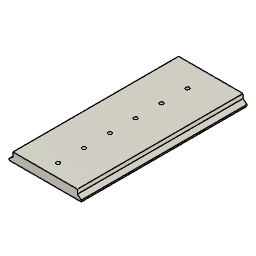
Fan Mount 50mm - BLANK_OLDV3_0 (Autodesk Fusion 360 design; units mm, degrees)
Autodesk Fusion 360 part; units mm, degrees
sketch "Sketch1" plane through (0, 0, 0) normal (0, 0, 1) x (1, 0, 0)
  line L0 (-27.9, 64) -> (27.9, 64)
  line L1 (27.9, 64) -> (27.9, -64)
  line L2 (27.9, -64) -> (-27.9, -64)
  line L3 (-27.9, -64) -> (-27.9, 64)
  line L4 (0, 76.2027) -> (0, 75)
  line L5 (0, 75) -> (0, -75) construction
  line L6 (-56.392, 0) -> (-53.853, 0)
  line L7 (-53.853, 0) -> (53.853, 0) construction
  point P0 (0, 64)
  point P1 (-27.9, 0)
  dimension "d44" = 150
  dimension "d45" = 128
  dimension "d46" = 55.8
  constraint horizontal L0
  constraint vertical L1
  constraint horizontal L2
  constraint vertical L3
  constraint midpoint L0 P0
  constraint midpoint L3 P1
  constraint vertical L4
  constraint parallel L4 L5
  constraint midpoint origin L5
  constraint perpendicular L3 L6
  constraint perpendicular L1 L7
  constraint midpoint origin L7
  constraint coincident P1 L7
  constraint coincident P0 L5
  measures "d44" distance of L4.end L5.end
  measures "d45" distance of L0.start L2.end
  measures "d46" distance of L0.start L0.end
extrude "Extrude1" add sketch "Sketch1" along normal blind 7
sketch "Sketch2" plane through (0, -64, 0) normal (0, -1, 0) x (1, 0, 0)
  line L0 (-27.9, 0) -> (27.9, 0)
  line L1 (27.9, 0) -> (27.9, 7)
  line L2 (27.9, 7) -> (-27.9, 7)
  line L3 (-27.9, 7) -> (-27.9, 0)
  line L4 (-27.9, 1.153) -> (-24.9009, 3.6695)
  line L5 (-24.9009, 3.6695) -> (-24.9009, 7)
  line L6 (27.9, 1.153) -> (24.9009, 3.6695)
  line L7 (24.9009, 3.6695) -> (24.9009, 7)
  dimension "d49" = 1.153
  dimension "d50" = 3.915
  dimension "d51" = 40
  dimension "d52" = 1.153
  dimension "d54" = 3.915
  dimension "d55" = 40
  constraint coincident L3 L4.start
  constraint coincident L2 L5.end
  constraint perpendicular L2 L5
  constraint coincident L1 L6.start
  constraint coincident L2 L7.end
  constraint perpendicular L2 L7
  measures "d49" distance of L0.start L4.start
  measures "d50" distance of L4.start L4.end
  measures "d51" angle of L0 L4
  measures "d52" distance of L0.end L6.start
  measures "d54" distance of L6.start L6.end
  measures "d55" angle of L0 L6
extrude "Extrude2" cut sketch "Sketch2" against normal through all contours L2 L3 L4 L5 | L1 L2 L6 L7
sketch "Sketch3" plane through (0, 0, 0) normal (0, 0, -1) x (1, 0, 0)
  line L0 (27.9, 64) -> (-27.9, 64)
  line L1 (-27.9, 64) -> (-27.9, -64)
  line L2 (-27.9, -64) -> (27.9, -64)
  line L3 (27.9, -64) -> (27.9, 64)
  line L4 (0, 64) -> (0, -64) construction
  circle A0 centre (0, 54) radius 1.425
  dimension "d57" = 2.85
  dimension "d58" = 10
  constraint midpoint L0 L4.start
  constraint midpoint L2 L4.end
  constraint coincident L4 A0.centre
  measures "d57" diameter of A0
  measures "d58" distance of L0 A0.centre
extrude "Extrude3" cut sketch "Sketch3" against normal blind 7 contours A0
pattern_linear "R-Pattern1" count 1 spacing 0 along (-1, 0, 0) count 6 spacing 20 along (0, 1, 0) of "Extrude3"
equation "d52 = d49"
equation "d54 = d50"
equation "d55 = d51"
